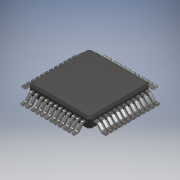
# Autodesk Inventor part: 24_pin_IC
Saved by Autodesk Inventor 2017 SP1 (Build 210196100, 196)
## iProperties
Created: 2016-08-29
Part Number: 24_pin_IC
Material: PBT Plastic
Document SubType Name: Modeling
Designer: jwrjc
Density: 1.31 g/cm^3
Appearance: Smooth - White
Author: jwrjc
Autodesk Inventor part; units mm, degrees
ref_plane "YZ Plane" through (0, 0, 0) normal (1, 0, 0) x (0, 1, 0)
ref_plane "XZ Plane" through (0, 0, 0) normal (0, 1, 0) x (-1, 0, 0)
ref_plane "XY Plane" through (0, 0, 0) normal (0, 0, 1) x (1, 0, 0)
sketch "Sketch1" plane through (0, 0, 0) normal (0, 0, 1) x (1, 0, 0)
  line L0 (-3.384, 5.7275) -> (-9.4565, 5.7275)
  line L1 (-9.7565, 5.4275) -> (-9.7565, -0.6228)
  line L2 (-9.4565, -0.9228) -> (-3.384, -0.9228)
  line L3 (-3.084, -0.6228) -> (-3.084, 5.4275)
  line L4 (-3.384, 5.7275) -> (-3.084, 5.4275)
  line L5 (-3.084, -0.6228) -> (-3.384, -0.9228)
  line L6 (-9.4565, -0.9228) -> (-9.7565, -0.6228)
  line L7 (-9.4565, 5.7275) -> (-9.7565, 5.4275)
  line L8 (-3.7705, 5.7275) -> (-3.5205, 5.7275)
  line L9 (-3.5205, 5.7275) -> (-3.5205, 7.1273)
  line L10 (-3.5205, 7.1273) -> (-3.7705, 7.1273)
  line L11 (-3.7705, 7.1273) -> (-3.7705, 5.7275)
  line L12 (-4.279, 5.7275) -> (-4.029, 5.7275)
  line L13 (-4.029, 5.7275) -> (-4.029, 7.1273)
  line L14 (-4.029, 7.1273) -> (-4.279, 7.1273)
  line L15 (-4.279, 7.1273) -> (-4.279, 5.7275)
  line L16 (-4.7309, 5.7275) -> (-4.4809, 5.7275)
  line L17 (-4.4809, 5.7275) -> (-4.4809, 7.1273)
  line L18 (-4.4809, 7.1273) -> (-4.7309, 7.1273)
  line L19 (-4.7309, 7.1273) -> (-4.7309, 5.7275)
  line L20 (-5.2394, 5.7275) -> (-4.9894, 5.7275)
  line L21 (-4.9894, 5.7275) -> (-4.9894, 7.1273)
  line L22 (-4.9894, 7.1273) -> (-5.2394, 7.1273)
  line L23 (-5.2394, 7.1273) -> (-5.2394, 5.7275)
  line L24 (-5.7196, 5.7275) -> (-5.4696, 5.7275)
  line L25 (-5.4696, 5.7275) -> (-5.4696, 7.1273)
  line L26 (-5.4696, 7.1273) -> (-5.7196, 7.1273)
  line L27 (-5.7196, 7.1273) -> (-5.7196, 5.7275)
  line L28 (-6.1716, 5.7275) -> (-5.9216, 5.7275)
  line L29 (-5.9216, 5.7275) -> (-5.9216, 7.1273)
  line L30 (-5.9216, 7.1273) -> (-6.1716, 7.1273)
  line L31 (-6.1716, 7.1273) -> (-6.1716, 5.7275)
  line L32 (-6.6703, 5.7275) -> (-6.4203, 5.7275)
  line L33 (-6.4203, 5.7275) -> (-6.4203, 7.1273)
  line L34 (-6.4203, 7.1273) -> (-6.6703, 7.1273)
  line L35 (-6.6703, 7.1273) -> (-6.6703, 5.7275)
  line L36 (-7.1745, 5.7275) -> (-6.9245, 5.7275)
  line L37 (-6.9245, 5.7275) -> (-6.9245, 7.1273)
  line L38 (-6.9245, 7.1273) -> (-7.1745, 7.1273)
  line L39 (-7.1745, 7.1273) -> (-7.1745, 5.7275)
  line L40 (-7.6688, 5.7275) -> (-7.4188, 5.7275)
  line L41 (-7.4188, 5.7275) -> (-7.4188, 7.1273)
  line L42 (-7.4188, 7.1273) -> (-7.6688, 7.1273)
  line L43 (-7.6688, 7.1273) -> (-7.6688, 5.7275)
  line L44 (-8.1491, 5.7275) -> (-7.8991, 5.7275)
  line L45 (-7.8991, 5.7275) -> (-7.8991, 7.1273)
  line L46 (-7.8991, 7.1273) -> (-8.1491, 7.1273)
  line L47 (-8.1491, 7.1273) -> (-8.1491, 5.7275)
  line L48 (-8.7423, 5.7275) -> (-8.4923, 5.7275)
  line L49 (-8.4923, 5.7275) -> (-8.4923, 7.1273)
  line L50 (-8.4923, 7.1273) -> (-8.7423, 7.1273)
  line L51 (-8.7423, 7.1273) -> (-8.7423, 5.7275)
  line L52 (-9.2508, 5.7275) -> (-9.0008, 5.7275)
  line L53 (-9.0008, 5.7275) -> (-9.0008, 7.1273)
  line L54 (-9.0008, 7.1273) -> (-9.2508, 7.1273)
  line L55 (-9.2508, 7.1273) -> (-9.2508, 5.7275)
  line L56 (-3.084, 2.4023) -> (-9.7565, 2.4023) construction
  line L57 (-6.4203, -0.9228) -> (-6.4203, 5.7275) construction
  line L58 (-3.7705, -0.9228) -> (-3.5205, -0.9228)
  line L59 (-3.5205, -0.9228) -> (-3.5205, -2.3226)
  line L60 (-3.5205, -2.3226) -> (-3.7705, -2.3226)
  line L61 (-3.7705, -2.3226) -> (-3.7705, -0.9228)
  line L62 (-4.279, -0.9228) -> (-4.029, -0.9228)
  line L63 (-4.029, -0.9228) -> (-4.029, -2.3226)
  line L64 (-4.029, -2.3226) -> (-4.279, -2.3226)
  line L65 (-4.279, -2.3226) -> (-4.279, -0.9228)
  line L66 (-4.7309, -0.9228) -> (-4.4809, -0.9228)
  line L67 (-4.4809, -0.9228) -> (-4.4809, -2.3226)
  line L68 (-4.4809, -2.3226) -> (-4.7309, -2.3226)
  line L69 (-4.7309, -2.3226) -> (-4.7309, -0.9228)
  line L70 (-5.2394, -0.9228) -> (-4.9894, -0.9228)
  line L71 (-4.9894, -0.9228) -> (-4.9894, -2.3226)
  line L72 (-4.9894, -2.3226) -> (-5.2394, -2.3226)
  line L73 (-5.2394, -2.3226) -> (-5.2394, -0.9228)
  line L74 (-5.7196, -0.9228) -> (-5.4696, -0.9228)
  line L75 (-5.4696, -0.9228) -> (-5.4696, -2.3226)
  line L76 (-5.4696, -2.3226) -> (-5.7196, -2.3226)
  line L77 (-5.7196, -2.3226) -> (-5.7196, -0.9228)
  line L78 (-6.1716, -0.9228) -> (-5.9216, -0.9228)
  line L79 (-5.9216, -0.9228) -> (-5.9216, -2.3226)
  line L80 (-5.9216, -2.3226) -> (-6.1716, -2.3226)
  line L81 (-6.1716, -2.3226) -> (-6.1716, -0.9228)
  line L82 (-6.6703, -0.9228) -> (-6.4203, -0.9228)
  line L83 (-6.4203, -0.9228) -> (-6.4203, -2.3226)
  line L84 (-6.4203, -2.3226) -> (-6.6703, -2.3226)
  line L85 (-6.6703, -2.3226) -> (-6.6703, -0.9228)
  line L86 (-7.1745, -0.9228) -> (-6.9245, -0.9228)
  line L87 (-6.9245, -0.9228) -> (-6.9245, -2.3226)
  line L88 (-6.9245, -2.3226) -> (-7.1745, -2.3226)
  line L89 (-7.1745, -2.3226) -> (-7.1745, -0.9228)
  line L90 (-7.6688, -0.9228) -> (-7.4188, -0.9228)
  line L91 (-7.4188, -0.9228) -> (-7.4188, -2.3226)
  line L92 (-7.4188, -2.3226) -> (-7.6688, -2.3226)
  line L93 (-7.6688, -2.3226) -> (-7.6688, -0.9228)
  line L94 (-8.1491, -0.9228) -> (-7.8991, -0.9228)
  line L95 (-7.8991, -0.9228) -> (-7.8991, -2.3226)
  line L96 (-7.8991, -2.3226) -> (-8.1491, -2.3226)
  line L97 (-8.1491, -2.3226) -> (-8.1491, -0.9228)
  line L98 (-8.7423, -0.9228) -> (-8.4923, -0.9228)
  line L99 (-8.4923, -0.9228) -> (-8.4923, -2.3226)
  line L100 (-8.4923, -2.3226) -> (-8.7423, -2.3226)
  line L101 (-8.7423, -2.3226) -> (-8.7423, -0.9228)
  line L102 (-9.2508, -0.9228) -> (-9.0008, -0.9228)
  line L103 (-9.0008, -0.9228) -> (-9.0008, -2.3226)
  line L104 (-9.0008, -2.3226) -> (-9.2508, -2.3226)
  line L105 (-9.2508, -2.3226) -> (-9.2508, -0.9228)
  line L106 (-3.084, 5.3232) -> (-1.4696, 5.3232)
  line L107 (-1.4696, 5.3232) -> (-1.4696, 5.0167)
  line L108 (-1.4696, 5.0167) -> (-3.084, 5.0167)
  line L109 (-3.084, 5.0167) -> (-3.084, 5.3232)
  line L110 (-3.084, 4.8231) -> (-1.4696, 4.8231)
  line L111 (-1.4696, 4.8231) -> (-1.4696, 4.5166)
  line L112 (-1.4696, 4.5166) -> (-3.084, 4.5166)
  line L113 (-3.084, 4.5166) -> (-3.084, 4.8231)
  line L114 (-3.084, 4.3311) -> (-1.4696, 4.3311)
  line L115 (-1.4696, 4.3311) -> (-1.4696, 4.0246)
  line L116 (-1.4696, 4.0246) -> (-3.084, 4.0246)
  line L117 (-3.084, 4.0246) -> (-3.084, 4.3311)
  line L118 (-3.084, 3.8229) -> (-1.4696, 3.8229)
  line L119 (-1.4696, 3.8229) -> (-1.4696, 3.5164)
  line L120 (-1.4696, 3.5164) -> (-3.084, 3.5164)
  line L121 (-3.084, 3.5164) -> (-3.084, 3.8229)
  line L122 (-3.084, 3.3228) -> (-1.4696, 3.3228)
  line L123 (-1.4696, 3.3228) -> (-1.4696, 3.0163)
  line L124 (-1.4696, 3.0163) -> (-3.084, 3.0163)
  line L125 (-3.084, 3.0163) -> (-3.084, 3.3228)
  line L126 (-3.084, 2.8066) -> (-1.4696, 2.8066)
  line L127 (-1.4696, 2.8066) -> (-1.4696, 2.5001)
  line L128 (-1.4696, 2.5001) -> (-3.084, 2.5001)
  line L129 (-3.084, 2.5001) -> (-3.084, 2.8066)
  line L130 (-3.084, 2.2985) -> (-1.4696, 2.2985)
  line L131 (-1.4696, 2.2985) -> (-1.4696, 1.992)
  line L132 (-1.4696, 1.992) -> (-3.084, 1.992)
  line L133 (-3.084, 1.992) -> (-3.084, 2.2985)
  line L134 (-3.084, 1.8306) -> (-1.4696, 1.8306)
  line L135 (-1.4696, 1.8306) -> (-1.4696, 1.5241)
  line L136 (-1.4696, 1.5241) -> (-3.084, 1.5241)
  line L137 (-3.084, 1.5241) -> (-3.084, 1.8306)
  line L138 (-3.084, 1.3305) -> (-1.4696, 1.3305)
  line L139 (-1.4696, 1.3305) -> (-1.4696, 1.0235)
  line L140 (-1.4696, 1.0235) -> (-3.084, 1.0235)
  line L141 (-3.084, 1.0235) -> (-3.084, 1.3305)
  line L142 (-3.084, 0.8466) -> (-1.4696, 0.8466)
  line L143 (-1.4696, 0.8466) -> (-1.4696, 0.5401)
  line L144 (-1.4696, 0.5401) -> (-3.084, 0.5401)
  line L145 (-3.084, 0.5401) -> (-3.084, 0.8466)
  line L146 (-3.084, 0.3465) -> (-1.4696, 0.3465)
  line L147 (-1.4696, 0.3465) -> (-1.4696, 0.0395)
  line L148 (-1.4696, 0.0395) -> (-3.084, 0.0395)
  line L149 (-3.084, 0.0395) -> (-3.084, 0.3465)
  line L150 (-3.084, -0.1536) -> (-1.4696, -0.1536)
  line L151 (-1.4696, -0.1536) -> (-1.4696, -0.4601)
  line L152 (-1.4696, -0.4601) -> (-3.084, -0.4601)
  line L153 (-3.084, -0.4601) -> (-3.084, -0.1536)
  line L154 (-9.7565, 5.3232) -> (-11.3709, 5.3232)
  line L155 (-11.3709, 5.3232) -> (-11.3709, 5.0167)
  line L156 (-11.3709, 5.0167) -> (-9.7565, 5.0167)
  line L157 (-9.7565, 4.8231) -> (-11.3709, 4.8231)
  line L158 (-11.3709, 4.8231) -> (-11.3709, 4.5166)
  line L159 (-11.3709, 4.5166) -> (-9.7565, 4.5166)
  line L160 (-9.7565, 4.3311) -> (-11.3709, 4.3311)
  line L161 (-11.3709, 4.3311) -> (-11.3709, 4.0246)
  line L162 (-11.3709, 4.0246) -> (-9.7565, 4.0246)
  line L163 (-9.7565, 3.8229) -> (-11.3709, 3.8229)
  line L164 (-11.3709, 3.8229) -> (-11.3709, 3.5164)
  line L165 (-11.3709, 3.5164) -> (-9.7565, 3.5164)
  line L166 (-9.7565, 3.3228) -> (-11.3709, 3.3228)
  line L167 (-11.3709, 3.3228) -> (-11.3709, 3.0163)
  line L168 (-11.3709, 3.0163) -> (-9.7565, 3.0163)
  line L169 (-9.7565, 2.8066) -> (-11.3709, 2.8066)
  line L170 (-11.3709, 2.8066) -> (-11.3709, 2.5001)
  line L171 (-11.3709, 2.5001) -> (-9.7565, 2.5001)
  line L172 (-9.7565, 2.2985) -> (-11.3709, 2.2985)
  line L173 (-11.3709, 2.2985) -> (-11.3709, 1.992)
  line L174 (-11.3709, 1.992) -> (-9.7565, 1.992)
  line L175 (-9.7565, 1.8306) -> (-11.3709, 1.8306)
  line L176 (-11.3709, 1.8306) -> (-11.3709, 1.5241)
  line L177 (-11.3709, 1.5241) -> (-9.7565, 1.5241)
  line L178 (-9.7565, 1.3305) -> (-11.3709, 1.3305)
  line L179 (-11.3709, 1.3305) -> (-11.3709, 1.0235)
  line L180 (-11.3709, 1.0235) -> (-9.7565, 1.0235)
  line L181 (-9.7565, 0.8466) -> (-11.3709, 0.8466)
  line L182 (-11.3709, 0.8466) -> (-11.3709, 0.5401)
  line L183 (-11.3709, 0.5401) -> (-9.7565, 0.5401)
  line L184 (-9.7565, 0.3465) -> (-11.3709, 0.3465)
  line L185 (-11.3709, 0.3465) -> (-11.3709, 0.0395)
  line L186 (-11.3709, 0.0395) -> (-9.7565, 0.0395)
  line L187 (-9.7565, -0.1536) -> (-11.3709, -0.1536)
  line L188 (-11.3709, -0.1536) -> (-11.3709, -0.4601)
  line L189 (-11.3709, -0.4601) -> (-9.7565, -0.4601)
  line L190 (-1.4696, 5.3232) -> (-3.084, 5.3232)
  line L191 (-3.084, 5.3232) -> (-3.084, 5.0167)
  line L192 (-3.084, 5.0167) -> (-1.4696, 5.0167)
  line L193 (-1.4696, 5.0167) -> (-1.4696, 5.3232)
  line L194 (-3.084, 4.8231) -> (-1.4696, 4.8231)
  line L195 (-1.4696, 4.8231) -> (-1.4696, 4.5166)
  line L196 (-1.4696, 4.5166) -> (-3.084, 4.5166)
  line L197 (-3.084, 4.5166) -> (-3.084, 4.8231)
  line L198 (-1.4696, 4.3311) -> (-3.084, 4.3311)
  line L199 (-3.084, 4.3311) -> (-3.084, 4.0246)
  line L200 (-3.084, 4.0246) -> (-1.4696, 4.0246)
  line L201 (-1.4696, 4.0246) -> (-1.4696, 4.3311)
  line L202 (-1.4696, 3.8229) -> (-3.084, 3.8229)
  line L203 (-3.084, 3.8229) -> (-3.084, 3.5164)
  line L204 (-3.084, 3.5164) -> (-1.4696, 3.5164)
  line L205 (-1.4696, 3.5164) -> (-1.4696, 3.8229)
  line L206 (-1.4696, 3.3228) -> (-3.084, 3.3228)
  line L207 (-3.084, 3.3228) -> (-3.084, 3.0163)
  line L208 (-3.084, 3.0163) -> (-1.4696, 3.0163)
  line L209 (-1.4696, 3.0163) -> (-1.4696, 3.3228)
  line L210 (-1.4696, 2.8066) -> (-3.084, 2.8066)
  line L211 (-3.084, 2.8066) -> (-3.084, 2.5001)
  line L212 (-3.084, 2.5001) -> (-1.4696, 2.5001)
  line L213 (-1.4696, 2.5001) -> (-1.4696, 2.8066)
  line L214 (-1.4696, 2.2985) -> (-3.084, 2.2985)
  line L215 (-3.084, 2.2985) -> (-3.084, 1.992)
  line L216 (-3.084, 1.992) -> (-1.4696, 1.992)
  line L217 (-1.4696, 1.992) -> (-1.4696, 2.2985)
  line L218 (-1.4696, 1.8306) -> (-3.084, 1.8306)
  line L219 (-3.084, 1.8306) -> (-3.084, 1.5241)
  line L220 (-3.084, 1.5241) -> (-1.4696, 1.5241)
  line L221 (-1.4696, 1.5241) -> (-1.4696, 1.8306)
  line L222 (-1.4696, 1.3305) -> (-3.084, 1.3305)
  line L223 (-3.084, 1.3305) -> (-3.084, 1.0235)
  line L224 (-3.084, 1.0235) -> (-1.4696, 1.0235)
  line L225 (-1.4696, 1.0235) -> (-1.4696, 1.3305)
  line L226 (-1.4696, 0.8466) -> (-3.084, 0.8466)
  line L227 (-3.084, 0.8466) -> (-3.084, 0.5401)
  line L228 (-3.084, 0.5401) -> (-1.4696, 0.5401)
  line L229 (-1.4696, 0.5401) -> (-1.4696, 0.8466)
  line L230 (-1.4696, 0.3465) -> (-3.084, 0.3465)
  line L231 (-3.084, 0.3465) -> (-3.084, 0.0395)
  line L232 (-3.084, 0.0395) -> (-1.4696, 0.0395)
  line L233 (-1.4696, 0.0395) -> (-1.4696, 0.3465)
  line L234 (-1.4696, -0.1536) -> (-3.084, -0.1536)
  line L235 (-3.084, -0.1536) -> (-3.084, -0.4601)
  line L236 (-3.084, -0.4601) -> (-1.4696, -0.4601)
  line L237 (-1.4696, -0.4601) -> (-1.4696, -0.1536)
  line L238 (-11.3709, -0.1536) -> (-9.7565, -0.1536)
  line L239 (-9.7565, -0.1536) -> (-9.7565, -0.4601)
  line L240 (-9.7565, -0.4601) -> (-11.3709, -0.4601)
  line L241 (-11.3709, -0.4601) -> (-11.3709, -0.1536)
  line L242 (-9.7565, 0.0395) -> (-11.3709, 0.0395)
  line L243 (-11.3709, 0.0395) -> (-11.3709, 0.3465)
  line L244 (-11.3709, 0.3465) -> (-9.7565, 0.3465)
  line L245 (-9.7565, 0.3465) -> (-9.7565, 0.0395)
  line L246 (-11.3709, 0.5401) -> (-9.7565, 0.5401)
  line L247 (-9.7565, 0.5401) -> (-9.7565, 0.8466)
  line L248 (-9.7565, 0.8466) -> (-11.3709, 0.8466)
  line L249 (-11.3709, 0.8466) -> (-11.3709, 0.5401)
  line L250 (-9.7565, 1.0235) -> (-11.3709, 1.0235)
  line L251 (-11.3709, 1.0235) -> (-11.3709, 1.3305)
  line L252 (-11.3709, 1.3305) -> (-9.7565, 1.3305)
  line L253 (-9.7565, 1.3305) -> (-9.7565, 1.0235)
  line L254 (-11.3709, 1.5241) -> (-9.7565, 1.5241)
  line L255 (-9.7565, 1.5241) -> (-9.7565, 1.8306)
  line L256 (-9.7565, 1.8306) -> (-11.3709, 1.8306)
  line L257 (-11.3709, 1.8306) -> (-11.3709, 1.5241)
  line L258 (-9.7565, 1.992) -> (-11.3709, 1.992)
  line L259 (-11.3709, 1.992) -> (-11.3709, 2.2985)
  line L260 (-11.3709, 2.2985) -> (-9.7565, 2.2985)
  line L261 (-9.7565, 2.2985) -> (-9.7565, 1.992)
  line L262 (-9.7565, 2.5001) -> (-11.3709, 2.5001)
  line L263 (-11.3709, 2.5001) -> (-11.3709, 2.8066)
  line L264 (-11.3709, 2.8066) -> (-9.7565, 2.8066)
  line L265 (-9.7565, 2.8066) -> (-9.7565, 2.5001)
  line L266 (-11.3709, 3.0163) -> (-9.7565, 3.0163)
  line L267 (-9.7565, 3.0163) -> (-9.7565, 3.3228)
  line L268 (-9.7565, 3.3228) -> (-11.3709, 3.3228)
  line L269 (-11.3709, 3.3228) -> (-11.3709, 3.0163)
  line L270 (-9.7565, 3.5164) -> (-11.3709, 3.5164)
  line L271 (-11.3709, 3.5164) -> (-11.3709, 3.8229)
  line L272 (-11.3709, 3.8229) -> (-9.7565, 3.8229)
  line L273 (-9.7565, 3.8229) -> (-9.7565, 3.5164)
  line L274 (-11.3709, 4.0246) -> (-9.7565, 4.0246)
  line L275 (-9.7565, 4.0246) -> (-9.7565, 4.3311)
  line L276 (-9.7565, 4.3311) -> (-11.3709, 4.3311)
  line L277 (-11.3709, 4.3311) -> (-11.3709, 4.0246)
  line L278 (-9.7565, 4.5166) -> (-11.3709, 4.5166)
  line L279 (-11.3709, 4.5166) -> (-11.3709, 4.8231)
  line L280 (-11.3709, 4.8231) -> (-9.7565, 4.8231)
  line L281 (-9.7565, 4.8231) -> (-9.7565, 4.5166)
  line L282 (-11.3709, 5.0167) -> (-9.7565, 5.0167)
  line L283 (-9.7565, 5.0167) -> (-9.7565, 5.3232)
  line L284 (-9.7565, 5.3232) -> (-11.3709, 5.3232)
  line L285 (-11.3709, 5.3232) -> (-11.3709, 5.0167)
  line L286 (-3.5205, -0.9228) -> (-3.7705, -0.9228)
  line L287 (-3.7705, -0.9228) -> (-3.7705, -2.3226)
  line L288 (-3.7705, -2.3226) -> (-3.5205, -2.3226)
  line L289 (-3.5205, -2.3226) -> (-3.5205, -0.9228)
  line L290 (-4.029, -2.3226) -> (-4.279, -2.3226)
  line L291 (-4.279, -2.3226) -> (-4.279, -0.9228)
  line L292 (-4.279, -0.9228) -> (-4.029, -0.9228)
  line L293 (-4.029, -0.9228) -> (-4.029, -2.3226)
  line L294 (-4.4809, -0.9228) -> (-4.7309, -0.9228)
  line L295 (-4.7309, -0.9228) -> (-4.7309, -2.2697)
  line L296 (-4.7309, -2.2697) -> (-4.4809, -2.2697)
  line L297 (-4.4809, -2.2697) -> (-4.4809, -0.9228)
  line L298 (-4.9894, -2.3226) -> (-5.2394, -2.3226)
  line L299 (-5.2394, -2.3226) -> (-5.2394, -0.9228)
  line L300 (-5.2394, -0.9228) -> (-4.9894, -0.9228)
  line L301 (-4.9894, -0.9228) -> (-4.9894, -2.3226)
  line L302 (-5.4696, -0.9228) -> (-5.7196, -0.9228)
  line L303 (-5.7196, -0.9228) -> (-5.7196, -2.3226)
  line L304 (-5.7196, -2.3226) -> (-5.4696, -2.3226)
  line L305 (-5.4696, -2.3226) -> (-5.4696, -0.9228)
  line L306 (-5.9216, -2.3226) -> (-6.1716, -2.3226)
  line L307 (-6.1716, -2.3226) -> (-6.1716, -0.9228)
  line L308 (-6.1716, -0.9228) -> (-5.9216, -0.9228)
  line L309 (-5.9216, -0.9228) -> (-5.9216, -2.3226)
  line L310 (-6.4203, -0.9228) -> (-6.6703, -0.9228)
  line L311 (-6.6703, -0.9228) -> (-6.6703, -2.3226)
  line L312 (-6.6703, -2.3226) -> (-6.4203, -2.3226)
  line L313 (-6.4203, -2.3226) -> (-6.4203, -0.9228)
  line L314 (-6.9245, -2.3226) -> (-7.1745, -2.3226)
  line L315 (-7.1745, -2.3226) -> (-7.1745, -0.9228)
  line L316 (-7.1745, -0.9228) -> (-6.9245, -0.9228)
  line L317 (-6.9245, -0.9228) -> (-6.9245, -2.3226)
  line L318 (-7.4188, -0.9228) -> (-7.6688, -0.9228)
  line L319 (-7.6688, -0.9228) -> (-7.6688, -2.3226)
  line L320 (-7.6688, -2.3226) -> (-7.4188, -2.3226)
  line L321 (-7.4188, -2.3226) -> (-7.4188, -0.9228)
  line L322 (-7.8991, -2.3226) -> (-8.1491, -2.3226)
  line L323 (-8.1491, -2.3226) -> (-8.1491, -0.9228)
  line L324 (-8.1491, -0.9228) -> (-7.8991, -0.9228)
  line L325 (-7.8991, -0.9228) -> (-7.8991, -2.3226)
  line L326 (-8.4923, -0.9228) -> (-8.7423, -0.9228)
  line L327 (-8.7423, -0.9228) -> (-8.7423, -2.2697)
  line L328 (-8.7423, -2.2697) -> (-8.4923, -2.2697)
  line L329 (-8.4923, -2.2697) -> (-8.4923, -0.9228)
  line L330 (-9.0008, -2.3226) -> (-9.2508, -2.3226)
  line L331 (-9.2508, -2.3226) -> (-9.2508, -0.9228)
  line L332 (-9.2508, -0.9228) -> (-9.0008, -0.9228)
  line L333 (-9.0008, -0.9228) -> (-9.0008, -2.3226)
  line L334 (-3.5205, 5.7275) -> (-3.7705, 5.7275)
  line L335 (-3.7705, 5.7275) -> (-3.7705, 7.1273)
  line L336 (-3.7705, 7.1273) -> (-3.5205, 7.1273)
  line L337 (-3.5205, 7.1273) -> (-3.5205, 5.7275)
  line L338 (-4.029, 7.1273) -> (-4.279, 7.1273)
  line L339 (-4.279, 7.1273) -> (-4.279, 5.7275)
  line L340 (-4.279, 5.7275) -> (-4.029, 5.7275)
  line L341 (-4.029, 5.7275) -> (-4.029, 7.1273)
  line L342 (-4.4809, 5.7275) -> (-4.7309, 5.7275)
  line L343 (-4.7309, 5.7275) -> (-4.7309, 7.1273)
  line L344 (-4.7309, 7.1273) -> (-4.4809, 7.1273)
  line L345 (-4.4809, 7.1273) -> (-4.4809, 5.7275)
  line L346 (-4.9894, 7.1273) -> (-5.2394, 7.1273)
  line L347 (-5.2394, 7.1273) -> (-5.2394, 5.7275)
  line L348 (-5.2394, 5.7275) -> (-4.9894, 5.7275)
  line L349 (-4.9894, 5.7275) -> (-4.9894, 7.1273)
  line L350 (-5.4696, 5.7275) -> (-5.7196, 5.7275)
  line L351 (-5.7196, 5.7275) -> (-5.7196, 7.1273)
  line L352 (-5.7196, 7.1273) -> (-5.4696, 7.1273)
  line L353 (-5.4696, 7.1273) -> (-5.4696, 5.7275)
  line L354 (-5.9216, 7.1273) -> (-6.1716, 7.1273)
  line L355 (-6.1716, 7.1273) -> (-6.1716, 5.7275)
  line L356 (-6.1716, 5.7275) -> (-5.9216, 5.7275)
  line L357 (-5.9216, 5.7275) -> (-5.9216, 7.1273)
  line L358 (-6.4203, 5.7275) -> (-6.6703, 5.7275)
  line L359 (-6.6703, 5.7275) -> (-6.6703, 7.1273)
  line L360 (-6.6703, 7.1273) -> (-6.4203, 7.1273)
  line L361 (-6.4203, 7.1273) -> (-6.4203, 5.7275)
  line L362 (-6.9245, 7.1273) -> (-7.1745, 7.1273)
  line L363 (-7.1745, 7.1273) -> (-7.1745, 5.7275)
  line L364 (-7.1745, 5.7275) -> (-6.9245, 5.7275)
  line L365 (-6.9245, 5.7275) -> (-6.9245, 7.1273)
  line L366 (-7.4188, 7.1273) -> (-7.6688, 7.1273)
  line L367 (-7.6688, 7.1273) -> (-7.6688, 5.7275)
  line L368 (-7.6688, 5.7275) -> (-7.4188, 5.7275)
  line L369 (-7.4188, 5.7275) -> (-7.4188, 7.1273)
  line L370 (-7.8991, 5.7275) -> (-8.1491, 5.7275)
  line L371 (-8.1491, 5.7275) -> (-8.1491, 7.1273)
  line L372 (-8.1491, 7.1273) -> (-7.8991, 7.1273)
  line L373 (-7.8991, 7.1273) -> (-7.8991, 5.7275)
  line L374 (-8.4923, 7.1273) -> (-8.7423, 7.1273)
  line L375 (-8.7423, 7.1273) -> (-8.7423, 5.7275)
  line L376 (-8.7423, 5.7275) -> (-8.4923, 5.7275)
  line L377 (-8.4923, 5.7275) -> (-8.4923, 7.1273)
  line L378 (-9.0008, 5.7275) -> (-9.2508, 5.7275)
  line L379 (-9.2508, 5.7275) -> (-9.2508, 7.1273)
  line L380 (-9.2508, 7.1273) -> (-9.0008, 7.1273)
  line L381 (-9.0008, 7.1273) -> (-9.0008, 5.7275)
  point P0 (0, 0)
  point P1 (-3.084, 5.7275)
  point P2 (-9.7565, -0.9228)
  point P3 (-9.7565, 5.7275)
  point P4 (-3.084, -0.9228)
  dimension "d0" = 0.3
  dimension "d1" = 0.3
  dimension "d2" = 0.3
  dimension "d3" = 0.3
  dimension "d4" = 0.3
  dimension "d5" = 0.3
  dimension "d6" = 0.3
  dimension "d7" = 0.3
  dimension "d8" = 0.25
  dimension "d9" = 0.25
  dimension "d10" = 0.25
  dimension "d11" = 0.25
  dimension "d12" = 0.25
  dimension "d13" = 0.25
  dimension "d14" = 0.25
  dimension "d15" = 0.25
  dimension "d16" = 0.25
  dimension "d17" = 0.25
  dimension "d18" = 0.25
  dimension "d19" = 0.25
  dimension "d20" = 0.307
  dimension "d21" = 0.307
  constraints: 760 end point, 144 parallel, 95 symmetric about line, 73 horizontal, 72 perpendicular, 51 point on line, 2 midpoint, 2 vertical, 35 other
  measures "d0" distance of L4.start point (-3.084, 5.727)
  measures "d1" distance of L4.end point (-3.084, 5.727)
  measures "d2" distance of L5.start point (-3.084, -0.923)
  measures "d3" distance of L2.end point (-3.084, -0.923)
  measures "d4" distance of L2.start point (-9.756, -0.923)
  measures "d5" distance of L1.end point (-9.756, -0.923)
  measures "d6" distance of L7.start point (-9.756, 5.727)
  measures "d7" distance of L1.start point (-9.756, 5.727)
  measures "d8" distance of L9.end L10.end
  measures "d9" distance of L13.end L14.end
  measures "d10" distance of L17.end L18.end
  measures "d11" distance of L21.end L22.end
  measures "d12" distance of L25.end L26.end
  measures "d13" distance of L29.end L30.end
  measures "d14" distance of L33.end L34.end
  measures "d15" distance of L37.end L38.end
  measures "d16" distance of L41.end L42.end
  measures "d17" distance of L45.end L46.end
  measures "d18" distance of L49.end L50.end
  measures "d19" distance of L53.end L54.end
  measures "d20" distance of L138.end L139.end
  measures "d21" distance of L146.end L147.end
extrude "Extrusion1" add sketch "Sketch1" along normal blind 1.2 contours L4 L3 L5 L2 L6 L1 L7 L0
extrude "Extrusion2" add sketch "Sketch1" along normal blind 0.8 separate body contours L0 L11 L10 L9 | L106 L107 L108 L3 | L0 L15 L14 L13 | L110 L111 L112 L3 | L0 L19 L18 L17 | L114 L115 L116 L3 | L0 L23 L22 L21 | L118 L119 L120 L3 | L0 L27 L26 L25 | L122 L123 L124 L3 | L0 L31 L30 L29 | L126 L127 L128 L3 | L0 L35 L34 L33 | L130 L131 L132 L3 | L0 L39 L38 L37 | L134 L135 L136 L3 | L0 L43 L42 L41 | L138 L139 L140 L3 | L0 L47 L46 L45 | L142 L143 L144 L3 | L0 L51 L50 L49 | L146 L147 L148 L3 | L0 L55 L54 L53 | L150 L151 L152 L3 | L1 L156 L155 L154 | L59 L60 L61 L2 | L1 L159 L158 L157 | L63 L64 L65 L2 | L1 L162 L161 L160 | L67 L296 L69 L2 | L1 L165 L164 L163 | L71 L72 L73 L2 | L1 L168 L167 L166 | L75 L76 L77 L2 | L1 L171 L170 L169 | L79 L80 L81 L2 | L1 L174 L173 L172 | L83 L84 L85 L2 | L1 L177 L176 L175 | L87 L88 L89 L2 | L1 L180 L179 L178 | L91 L92 L93 L2 | L1 L183 L182 L181 | L95 L96 L97 L2 | L1 L186 L185 L184 | L99 L328 L101 L2 | L1 L189 L188 L187 | L103 L104 L105 L2
chamfer "Chamfer1" distance 0.2 angle 45 70 edges at (-9.3536, 5.7275, 1.2) (-3.5772, 5.7275, 1.2) (-3.234, 5.5775, 1.2) (-3.084, 5.3753, 1.2) (-3.084, -0.3882, 1.2) (-3.234, -0.7728, 1.2) (-4.9021, -0.9228, 1.2) (-7.9384, -0.9228, 1.2) (-9.6065, -0.7728, 1.2) (-9.7565, 2.4023, 1.2) (-9.6065, 5.5775, 1.2) (-9.6065, -0.7728, 0) (-4.9021, -0.9228, 0) (-7.9384, -0.9228, 0) (-9.7565, 2.4023, 0) (-3.234, -0.7728, 0) (-3.084, 5.3753, 0) (-3.084, -0.3882, 0) (-9.6065, 5.5775, 0) (-9.3536, 5.7275, 0) (-3.5772, 5.7275, 0) (-3.234, 5.5775, 0) (-6.5453, -0.9228, 0) (-3.6455, -0.9228, 0) (-5.1144, -0.9228, 0) (-4.154, -0.9228, 0) (-5.5946, -0.9228, 0) (-6.0466, -0.9228, 0) (-7.0495, -0.9228, 0) (-7.5438, -0.9228, 0) (-8.0241, -0.9228, 0) (-9.1258, -0.9228, 0) (-4.6059, -0.9228, 0) (-8.6173, -0.9228, 0) (-9.7565, 5.1699, 0) (-9.7565, 4.6698, 0) (-9.7565, 4.1778, 0) (-9.7565, 3.6697, 0) (-9.7565, 3.1696, 0) (-9.7565, 2.6534, 0) (-9.7565, 2.1452, 0) (-9.7565, 0.6933, 0) (-9.7565, -0.3068, 0) (-9.7565, 1.6774, 0) (-9.7565, 0.193, 0) (-9.7565, 1.177, 0) (-3.084, 5.1699, 0) (-3.084, 4.6698, 0) (-3.084, 4.1778, 0) (-3.084, 3.6697, 0) (-3.084, 3.1696, 0) (-3.084, 2.6534, 0) (-3.084, 2.1452, 0) (-3.084, 1.6774, 0) (-3.084, 0.6933, 0) (-3.084, -0.3068, 0) (-3.084, 1.177, 0) (-3.084, 0.193, 0) (-9.1258, 5.7275, 0) (-8.6173, 5.7275, 0) (-8.0241, 5.7275, 0) (-7.5438, 5.7275, 0) (-7.0495, 5.7275, 0) (-6.5453, 5.7275, 0) (-6.0466, 5.7275, 0) (-5.5946, 5.7275, 0) (-5.1144, 5.7275, 0) (-4.6059, 5.7275, 0) (-4.154, 5.7275, 0) (-3.6455, 5.7275, 0)
sketch "Sketch2" plane through (-11.3709, -0.4601, 0) normal (0, -1, 0) x (1, 0, 0)
  line L0 (0, 0) -> (0, 0.8) projected
  line L1 (0, 0) -> (0, 0.8)
  line L2 (0, 0.8) -> (1.6144, 0.8) projected
  line L3 (0, 0.8) -> (1.6144, 0.8)
  line L4 (1.6144, 0.8) -> (1.6144, 0.6295)
  line L5 (1.6144, 0) -> (1.6144, 0.8) projected
  line L6 (1.3568, 0.6295) -> (0.9924, 0)
  line L7 (0, 0) -> (1.6144, 0) projected
  line L8 (1.3568, 0.6295) -> (1.6144, 0.6295)
  line L9 (0.9924, 0) -> (0.5324, 0)
  line L10 (0.5324, 0.1413) -> (0.9145, 0.1413)
  line L11 (0.9145, 0.1413) -> (1.2958, 0.8)
  line L12 (0.5324, 0.1413) -> (0.5324, 0)
  line L13 (1.2958, 0.8) -> (1.6144, 0.8)
  line L14 (1.6144, 0.6295) -> (1.6144, 0.8)
  line L15 (8.2869, 0.2) -> (8.2869, 1) projected
  line L16 (8.2869, 0.8) -> (8.6183, 0.8)
  line L17 (8.6183, 0.8) -> (9.1778, 0.1632)
  line L18 (9.1778, 0.1632) -> (9.5758, 0.1632)
  line L19 (9.5758, 0.1632) -> (9.5758, 0)
  line L20 (9.5758, 0) -> (9.1391, 0)
  line L21 (9.9013, 0) -> (8.2869, 0) projected
  line L22 (9.1391, 0) -> (8.5851, 0.6306)
  line L23 (8.5851, 0.6306) -> (8.2869, 0.6306)
  line L24 (8.2869, 0) -> (8.2869, 0.8) projected
  line L25 (8.2869, 0.6306) -> (8.2869, 0.8)
  line L26 (8.2869, 0.8) -> (8.2869, 0.6306)
  line L27 (9.9013, 0.8) -> (8.2869, 0.8) projected
  line L28 (8.6183, 0.8) -> (9.9013, 0.8)
  line L29 (9.9013, 0.8) -> (9.9013, 0)
  line L30 (0.5324, 0) -> (0, 0)
  line L31 (1.6144, 0) -> (1.6144, 0.6295)
  line L32 (8.2869, 0.6306) -> (8.5851, 0.6306)
  line L33 (9.1391, 0) -> (8.2869, 0)
  line L34 (8.2869, 0.6306) -> (8.2869, 0.8)
  line L35 (8.6183, 0.8) -> (8.2869, 0.8)
  point P0 (11.3709, 0)
  constraints: 56 end point, 9 collinear, 6 perpendicular, 5 parallel, 5 point on line, 2 horizontal, 1 vertical
extrude "Extrusion3" cut sketch "Sketch2" against normal blind 5.8 contours L0 L2 L11 L10 L12 L7 | L6 L8 L5 L7 | L15 L23 L22 L21 L24 | L27 L29 L21 L19 L18 L17 bodies 2
fillet "Fillet1" radius 0.2 96 edges at (-10.0751, 5.1699, 0.8) (-10.4564, 5.1699, 0.1413) (-10.0751, 4.6698, 0.8) (-10.4564, 4.6698, 0.1413) (-10.0751, 4.1778, 0.8) (-10.4564, 4.1778, 0.1413) (-10.0751, 3.6697, 0.8) (-10.4564, 3.6697, 0.1413) (-10.0751, 3.1696, 0.8) (-10.4564, 3.1696, 0.1413) (-10.0751, 2.6534, 0.8) (-10.4564, 2.6534, 0.1413) (-10.4564, 2.1452, 0.1413) (-10.0751, 2.1452, 0.8) (-10.0751, 1.6774, 0.8) (-10.4564, 1.6774, 0.1413) (-10.0751, 1.177, 0.8) (-10.4564, 1.177, 0.1413) (-10.0751, 0.6933, 0.8) (-10.4564, 0.6933, 0.1413) (-10.0751, 0.193, 0.8) (-10.4564, 0.193, 0.1413) (-10.4564, -0.3068, 0.1413) (-10.0751, -0.3068, 0.8) (-2.7526, 5.1699, 0.8) (-2.7526, 4.6698, 0.8) (-2.7526, 4.1778, 0.8) (-2.7526, 3.6697, 0.8) (-2.7526, 3.1696, 0.8) (-2.7526, 2.6534, 0.8) (-2.7526, 2.1452, 0.8) (-2.7526, 1.6774, 0.8) (-2.7526, 1.177, 0.8) (-2.7526, 0.6933, 0.8) (-2.7526, 0.193, 0.8) (-2.7526, -0.3068, 0.8) (-2.1931, -0.3068, 0.1632) (-2.1931, 0.193, 0.1632) (-2.1931, 0.6933, 0.1632) (-2.1931, 1.177, 0.1632) (-2.1931, 1.6774, 0.1632) (-2.1931, 2.1452, 0.1632) (-2.1931, 2.6534, 0.1632) (-2.1931, 3.1696, 0.1632) (-2.1931, 3.6697, 0.1632) (-2.1931, 4.1778, 0.1632) (-2.1931, 4.6698, 0.1632) (-2.1931, 5.1699, 0.1632) (-10.3785, -0.3068, 0) (-10.3785, 0.193, 0) (-10.3785, 0.6933, 0) (-10.3785, 1.177, 0) (-10.3785, 1.6774, 0) (-10.3785, 2.1452, 0) (-10.3785, 2.6534, 0) (-10.3785, 3.1696, 0) (-10.3785, 3.6697, 0) (-10.3785, 4.1778, 0) (-10.3785, 4.6698, 0) (-10.3785, 5.1699, 0) (-10.0141, 5.1699, 0.6295) (-10.0141, 4.6698, 0.6295) (-10.0141, 4.1778, 0.6295) (-10.0141, 3.6697, 0.6295) (-10.0141, 3.1696, 0.6295) (-10.0141, 2.6534, 0.6295) (-10.0141, 2.1452, 0.6295) (-10.0141, 1.6774, 0.6295) (-10.0141, 1.177, 0.6295) (-10.0141, 0.6933, 0.6295) (-10.0141, 0.193, 0.6295) (-10.0141, -0.3068, 0.6295) (-2.7858, -0.3068, 0.6306) (-2.7858, 0.193, 0.6306) (-2.7858, 0.6933, 0.6306) (-2.7858, 1.177, 0.6306) (-2.7858, 1.6774, 0.6306) (-2.7858, 2.1452, 0.6306) (-2.7858, 2.6534, 0.6306) (-2.7858, 3.1696, 0.6306) (-2.7858, 3.6697, 0.6306) (-2.7858, 4.1778, 0.6306) (-2.7858, 4.6698, 0.6306) (-2.7858, 5.1699, 0.6306) (-2.2318, 5.1699, 0) (-2.2318, 4.6698, 0) (-2.2318, 4.1778, 0) (-2.2318, 3.6697, 0) (-2.2318, 3.1696, 0) (-2.2318, 2.6534, 0) (-2.2318, 2.1452, 0) (-2.2318, 1.6774, 0) (-2.2318, 1.177, 0) (-2.2318, 0.6933, 0) (-2.2318, 0.193, 0) (-2.2318, -0.3068, 0)
sketch "Sketch3" plane through (-9.2508, 5.7275, 0) normal (-1, 0, 0) x (0, 0, 1)
  line L0 (0.8, 0) -> (0.8, 0.2722)
  line L1 (0.8, 0) -> (0.8, 1.3998) projected
  line L2 (0.8, 0.2722) -> (0.1493, 0.7639)
  line L3 (0.1493, 0.7639) -> (0.1493, 1.1547)
  line L4 (0.1493, 1.1547) -> (0, 1.1547)
  line L5 (0, 0) -> (0, 1.3998) projected
  line L6 (0, 0.6312) -> (0.5873, 0.1874)
  line L7 (0.5873, 0.1874) -> (0.5873, 0)
  line L8 (0, 0) -> (0.8, 0) projected
  line L9 (0.5873, 0) -> (0.6403, 0)
  line L10 (0.8, 0.2722) -> (0.8, 1.3998)
  line L11 (0, 1.3998) -> (0, 1.1547)
  line L12 (0, 0.6312) -> (0, 0)
  line L13 (0.5873, 0) -> (0.5873, 0.1874)
  line L14 (0.8, -6.6503) -> (0.8, -8.0501) projected
  line L15 (0.8, -6.6503) -> (0.8, -6.9122)
  line L16 (0.8, -6.9122) -> (0.1617, -7.4414)
  line L17 (0.1617, -7.4414) -> (0.1617, -7.8818)
  line L18 (0.1617, -7.8818) -> (0, -7.8818)
  line L19 (0, -7.8818) -> (0, -7.3535)
  line L20 (0, -7.3535) -> (0.6403, -6.8226)
  line L21 (0.6403, -6.8226) -> (0.6403, -6.6503)
  line L22 (0, -6.6503) -> (0.8, -6.6503) projected
  line L23 (0.6403, -6.6503) -> (0.8, -6.6503)
  line L24 (0, -8.0501) -> (0.8, -8.0501) projected
  line L25 (0.8, -6.6503) -> (0.8, -8.0501)
  line L26 (0.8, -8.0501) -> (0, -8.0501)
  line L27 (0, -8.0501) -> (0, -7.8818)
  line L28 (0, -6.6503) -> (0, -7.9972) projected
  line L29 (0, -7.3535) -> (0, -6.6503)
  line L30 (0, -6.6503) -> (0.6403, -6.6503)
  line L31 (0, 1.3998) -> (0.8, 1.3998)
  line L32 (0, 0) -> (0.5873, 0)
  line L33 (0.5873, 0.1874) -> (0.5873, 0)
  line L34 (0, 0) -> (0.5873, 0)
  line L35 (0, 0.6312) -> (0.5873, 0.1874)
  line L36 (0.6403, -6.6503) -> (0, -6.6503)
  line L37 (0, -7.3535) -> (0, -6.6503)
  line L38 (0.8, -6.9122) -> (0.8, -8.0501)
  line L39 (0.8, -8.0501) -> (0, -8.0501)
  line L40 (0, -7.8818) -> (0.1617, -7.8818)
  line L41 (0.8, -6.6503) -> (0, -6.6503)
  line L42 (0, -6.6503) -> (0, -8.0501)
  line L43 (0, -8.0501) -> (0.8, -8.0501)
  line L44 (0.8, -8.0501) -> (0.8, -6.6503)
  line L45 (0.8, 1.3998) -> (0, 1.3998)
  line L46 (0, 0) -> (0.5873, 0)
  line L47 (0.8, 0) -> (0.8, 1.3998)
  line L48 (0, 1.3998) -> (0, 1.1547)
  line L49 (0, 0.6312) -> (0, 0)
  point P0 (0, -5.7275)
  point P1 (0.8, 0.2722)
  constraints: 87 end point, 14 parallel, 14 perpendicular, 8 point on line, 7 collinear, 3 horizontal
extrude "Extrusion4" cut sketch "Sketch3" against normal blind 5.95 contours L2 L3 L4 L5 L31 L1 | L8 L5 L6 L7 | L14 L24 L27 L18 L17 L16 | L21 L20 L28 L22 bodies 2
fillet "Fillet2" radius 0.2 48 edges at (-3.6455, 6.4913, 0.1493) (-3.6455, 5.9997, 0.8) (-4.154, 5.9997, 0.8) (-4.154, 6.4913, 0.1493) (-4.6059, 6.4913, 0.1493) (-4.6059, 5.9997, 0.8) (-5.1144, 5.9997, 0.8) (-5.1144, 6.4913, 0.1493) (-5.5946, 6.4913, 0.1493) (-5.5946, 5.9997, 0.8) (-6.0466, 5.9997, 0.8) (-6.0466, 6.4913, 0.1493) (-6.5453, 6.4913, 0.1493) (-6.5453, 5.9997, 0.8) (-7.0495, 5.9997, 0.8) (-7.0495, 6.4913, 0.1493) (-7.5438, 6.4913, 0.1493) (-7.5438, 5.9997, 0.8) (-8.0241, 5.9997, 0.8) (-8.0241, 6.4913, 0.1493) (-8.6173, 5.9997, 0.8) (-8.6173, 6.4913, 0.1493) (-9.1258, 6.4913, 0.1493) (-9.1258, 5.9997, 0.8) (-3.6455, -1.7139, 0.1617) (-4.154, -1.7139, 0.1617) (-4.6059, -1.7139, 0.1617) (-5.1144, -1.7139, 0.1617) (-5.5946, -1.7139, 0.1617) (-6.0466, -1.7139, 0.1617) (-6.5453, -1.7139, 0.1617) (-7.0495, -1.7139, 0.1617) (-7.5438, -1.7139, 0.1617) (-8.0241, -1.7139, 0.1617) (-8.6173, -1.7139, 0.1617) (-9.1258, -1.7139, 0.1617) (-9.1258, -1.1847, 0.8) (-8.6173, -1.1847, 0.8) (-8.0241, -1.1847, 0.8) (-7.5438, -1.1847, 0.8) (-7.0495, -1.1847, 0.8) (-6.5453, -1.1847, 0.8) (-6.0466, -1.1847, 0.8) (-5.5946, -1.1847, 0.8) (-5.1144, -1.1847, 0.8) (-4.6059, -1.1847, 0.8) (-4.154, -1.1847, 0.8) (-3.6455, -1.1847, 0.8)
fillet "Fillet3" radius 0.2 48 edges at (-9.1258, 5.9149, 0.5873) (-9.1258, 6.3587, 0) (-8.6173, 6.3587, 0) (-8.6173, 5.9149, 0.5873) (-8.0241, 6.3587, 0) (-8.0241, 5.9149, 0.5873) (-7.5438, 6.3587, 0) (-7.5438, 5.9149, 0.5873) (-7.0495, 6.3587, 0) (-7.0495, 5.9149, 0.5873) (-6.5453, 6.3587, 0) (-6.5453, 5.9149, 0.5873) (-6.0466, 6.3587, 0) (-6.0466, 5.9149, 0.5873) (-5.5946, 6.3587, 0) (-5.5946, 5.9149, 0.5873) (-5.1144, 6.3587, 0) (-5.1144, 5.9149, 0.5873) (-4.6059, 6.3587, 0) (-4.6059, 5.9149, 0.5873) (-4.154, 6.3587, 0) (-4.154, 5.9149, 0.5873) (-3.6455, 6.3587, 0) (-3.6455, 5.9149, 0.5873) (-9.1258, -1.0951, 0.6403) (-8.6173, -1.0951, 0.6403) (-8.0241, -1.0951, 0.6403) (-7.5438, -1.0951, 0.6403) (-7.0495, -1.0951, 0.6403) (-6.5453, -1.0951, 0.6403) (-6.0466, -1.0951, 0.6403) (-5.5946, -1.0951, 0.6403) (-5.1144, -1.0951, 0.6403) (-4.6059, -1.0951, 0.6403) (-4.154, -1.0951, 0.6403) (-3.6455, -1.0951, 0.6403) (-3.6455, -1.626, 0) (-4.154, -1.626, 0) (-4.6059, -1.626, 0) (-5.1144, -1.626, 0) (-5.5946, -1.626, 0) (-6.0466, -1.626, 0) (-6.5453, -1.626, 0) (-7.0495, -1.626, 0) (-7.5438, -1.626, 0) (-8.0241, -1.626, 0) (-8.6173, -1.626, 0) (-9.1258, -1.626, 0)
equation "\"d1\" = d0"
equation "\"d2\" = d0"
equation "\"d3\" = d2"
equation "\"d4\" = d0"
equation "\"d5\" = d4"
equation "\"d6\" = d0"
equation "\"d7\" = d6"
body "Solid1"
body "Solid2"
